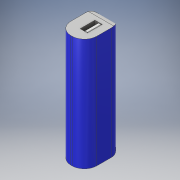
# Autodesk Inventor part: Powerbank
Saved by Autodesk Inventor 2018 (Build 220112000, 112)
## iProperties
Created: 2018-02-01
Part Number: Powerbank
Material: Generic
Document SubType Name: Modeling
Designer: Mandus
Density: 1 g/cm^3
Appearance: Default
Author: Mandus
Autodesk Inventor part; units mm, degrees
ref_plane "YZ Plane" through (0, 0, 0) normal (1, 0, 0) x (0, 1, 0)
ref_plane "XZ Plane" through (0, 0, 0) normal (0, 1, 0) x (-1, 0, 0)
ref_plane "XY Plane" through (0, 0, 0) normal (0, 0, 1) x (1, 0, 0)
sketch "Sketch1" plane through (0, 0, 0) normal (0, 1, 0) x (-1, 0, 0)
  line L0 (3.1776, 14.7647) -> (24.1776, 14.7647)
  line L1 (24.1776, 14.7647) -> (24.1776, -15.2353)
  line L2 (24.1776, -15.2353) -> (3.1776, -15.2353)
  line L3 (3.1776, -15.2353) -> (3.1776, 14.7647)
  dimension "d4" = 30
  dimension "d5" = 21
  constraints: 8 end point, 2 parallel, 1 horizontal, 1 perpendicular
  measures "d4" distance of L0.end L1.end
  measures "d5" distance of L1.end L2.end
extrude "Extrusion1" add sketch "Sketch1" along normal blind 91
fillet "Fillet1" radius 10 2 edges at (-3.1776, 45.5, 14.7647) (-24.1776, 45.5, 14.7647)
fillet "Fillet2" radius 6 2 edges at (-13.6776, 91, -15.2353) (-13.6776, 0, -15.2353)
sketch "Sketch2" plane through (0, 91, 0) normal (0, 1, 0) x (1, 0, 0)
  line L0 (-3.1776, 15.2353) -> (-3.1776, 7.2353)
  line L1 (-24.1776, 7.2353) -> (-24.1776, 15.2353)
  line L2 (-9.1776, 15.2353) -> (-3.1776, 15.2353)
  line L3 (-3.1776, 15.2353) -> (-3.1776, 7.2353)
  line L4 (-3.1776, 7.2353) -> (1.8224, 7.2353) construction
  arc A0 (-3.1776, 7.2353) -> (-9.1776, 15.2353) centre (-11.5109, 7.2353) ccw
  line L5 (-24.1776, 15.2353) -> (-18.1776, 15.2353)
  line L6 (-24.1776, 7.2353) -> (-24.1776, 15.2353)
  arc A1 (-18.1776, 15.2353) -> (-24.1776, 7.2353) centre (-15.8442, 7.2353) ccw
  line L7 (-24.1776, 15.2353) -> (-18.1776, 15.2353)
  line L8 (-3.1776, 15.2353) -> (-9.1776, 15.2353)
  point P0 (0, 0)
  dimension "d10" = 21
  dimension "d11" = 8
  dimension "d12" = 6
  dimension "d20" = 8
  dimension "d21" = 6
  constraints: 18 end point, 4 point on circle, 2 centre point, 2 horizontal, 1 parallel
  measures "d10" distance of L0.end L1.start
  measures "d11" distance of L0.start L0.end
  measures "d12" distance of L2.start L2.end
  measures "d20" distance of L1.start L1.end
  measures "d21" distance of L1.end L5.end
extrude "Extrusion3" cut sketch "Sketch2" against normal up to next
sketch "Sketch3" plane through (0, 91, 0) normal (0, 1, 0) x (1, 0, 0)
  line L0 (-9.1776, -6.2647) -> (-15.1776, -6.2647)
  line L1 (-15.1776, -6.2647) -> (-15.1776, 5.7353)
  line L2 (-15.1776, 5.7353) -> (-9.1776, 5.7353)
  line L3 (-9.1776, 5.7353) -> (-9.1776, -6.2647)
  line L4 (-3.1776, -4.7647) -> (-3.1776, 7.2353) projected
  line L5 (-14.1776, -14.7647) -> (-13.1776, -14.7647) projected
  point P0 (0, 0)
  dimension "d24" = 6
  dimension "d25" = 12
  dimension "d26" = 6
  dimension "d27" = 8.5
  constraints: 8 end point, 2 parallel, 1 horizontal, 1 perpendicular
  measures "d24" distance of L1.end L2.end
  measures "d25" distance of L0.end L1.end
  measures "d26" distance between parallel lines of L3 L4
  measures "d27" distance from line of L5 L0.end
sketch "Sketch4" plane through (0, 91, 0) normal (0, 1, 0) x (1, 0, 0)
  line L0 (-9.6776, -5.7647) -> (-11.6776, -5.7647)
  line L1 (-11.6776, -5.7647) -> (-11.6776, 5.2353)
  line L2 (-11.6776, 5.2353) -> (-9.6776, 5.2353)
  line L3 (-9.6776, 5.2353) -> (-9.6776, -5.7647)
  line L4 (-3.1776, -4.7647) -> (-3.1776, 7.2353) projected
  line L5 (-14.1776, -14.7647) -> (-13.1776, -14.7647) projected
  point P0 (0, 0)
  dimension "d28" = 2
  dimension "d29" = 11
  dimension "d30" = 6.5
  dimension "d31" = 9
  constraints: 8 end point, 2 parallel, 1 horizontal, 1 perpendicular
  measures "d28" distance of L0.start L0.end
  measures "d29" distance of L0.end L1.end
  measures "d30" distance from line of L4 L2.end
  measures "d31" distance from line of L5 L0.end
extrude "Extrusion4" cut sketch "Sketch3" against normal blind 10
extrude "Extrusion5" add sketch "Sketch4" against normal blind 10
sketch "Sketch5" plane through (0, 91, 0) normal (0, 1, 0) x (1, 0, 0)
  arc A0 (-13.1776, -14.7647) -> (-3.1776, -4.7647) centre (-13.1776, -4.7647) ccw projected
  line L0 (-14.1776, -14.7647) -> (-13.1776, -14.7647) projected
  arc A1 (-24.1776, -4.7647) -> (-14.1776, -14.7647) centre (-14.1776, -4.7647) ccw projected
  line L1 (-24.1776, 7.2353) -> (-24.1776, -4.7647) projected
  arc A2 (-23.934, 9.2353) -> (-24.1776, 7.2353) centre (-15.8442, 7.2353) ccw projected
  line L2 (-9.1776, 15.2353) -> (-18.1776, 15.2353) projected
  arc A3 (-3.1776, 7.2353) -> (-3.4211, 9.2353) centre (-11.5109, 7.2353) ccw projected
  line L3 (-3.1776, -4.7647) -> (-3.1776, 7.2353) projected
  line L4 (-9.1776, -6.2647) -> (-15.1776, -6.2647) projected
  line L5 (-9.1776, 5.7353) -> (-9.1776, -6.2647) projected
  line L6 (-15.1776, 5.7353) -> (-9.1776, 5.7353) projected
  line L7 (-15.1776, -6.2647) -> (-15.1776, 5.7353) projected
  point P0 (0, 0)
  constraints: 2 other
body "Solid1"
